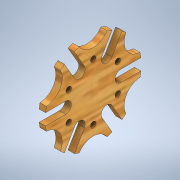
# Autodesk Inventor part: GenevaGear
Saved by Autodesk Inventor 2020.2 (Build 242310000, 310)
## iProperties
Created: 2019-12-15
Part Number: GenevaGear
Material: Plywood, Finish
Document SubType Name: Modeling
Designer: Paul Lefeuvre
Density: 0.552 g/cm^3
Appearance: Plywood - New
Author: Paul Lefeuvre
Autodesk Inventor part; units mm, degrees
ref_plane "YZ Plane" through (0, 0, 0) normal (1, 0, 0) x (0, 1, 0)
ref_plane "XZ Plane" through (0, 0, 0) normal (0, 1, 0) x (-1, 0, 0)
ref_plane "XY Plane" through (0, 0, 0) normal (0, 0, 1) x (1, 0, 0)
sketch "Sketch1" plane through (0, 0, 0) normal (1, 0, 0) x (0, 1, 0)
  circle A0 centre (0, 0) radius 100 construction
  circle A1 centre (0, 0) radius 72.5 construction
  circle A2 centre (0, 0) radius 110 construction
  circle A3 centre (0, 0) radius 67.7492
  line L0 (7.5, -38.8746) -> (7.5, -67.3328) construction
  line L1 (-7.5, -38.8746) -> (-7.5, -67.3328) construction
  arc A4 (7.5, -38.8746) -> (-7.5, -38.8746) centre (0, -38.8746) ccw construction
  line L2 (0, 0) -> (0, -136.3111) construction
  line L3 (8.1, -67.2632) -> (8.1, -38.8746)
  arc A5 (8.1, -38.8746) -> (-8.1, -38.8746) centre (0, -38.8746) ccw
  line L4 (-8.1, -38.8746) -> (-8.1, -67.2632)
  line L5 (62.3017, -26.6168) -> (37.7164, -12.4225)
  arc A6 (37.7164, -12.4225) -> (29.6164, -26.4521) centre (33.6664, -19.4373) ccw
  line L6 (29.6164, -26.4521) -> (54.2017, -40.6464)
  line L7 (54.2017, 40.6464) -> (29.6164, 26.4521)
  arc A7 (29.6164, 26.4521) -> (37.7164, 12.4225) centre (33.6664, 19.4373) ccw
  line L8 (37.7164, 12.4225) -> (62.3017, 26.6168)
  line L9 (-8.1, 67.2632) -> (-8.1, 38.8746)
  arc A8 (-8.1, 38.8746) -> (8.1, 38.8746) centre (0, 38.8746) ccw
  line L10 (8.1, 38.8746) -> (8.1, 67.2632)
  line L11 (-62.3017, 26.6168) -> (-37.7164, 12.4225)
  arc A9 (-37.7164, 12.4225) -> (-29.6164, 26.4521) centre (-33.6664, 19.4373) ccw
  line L12 (-29.6164, 26.4521) -> (-54.2017, 40.6464)
  line L13 (-54.2017, -40.6464) -> (-29.6164, -26.4521)
  arc A10 (-29.6164, -26.4521) -> (-37.7164, -12.4225) centre (-33.6664, -19.4373) ccw
  line L14 (-37.7164, -12.4225) -> (-62.3017, -26.6168)
  line L15 (37.4164, -12.9421) -> (62.0619, -27.1712) construction
  arc A11 (37.4164, -12.9421) -> (29.9164, -25.9325) centre (33.6664, -19.4373) ccw construction
  line L16 (29.9164, -25.9325) -> (54.5619, -40.1616) construction
  circle A12 centre (38.8746, -67.3328) radius 46.3746 construction
  circle A13 centre (38.8746, -67.3328) radius 31.3746 construction
  circle A14 centre (0, 0) radius 31.3746 construction
  arc A15 (49.513, -46.243) -> (15.2911, -66.001) centre (38.8746, -67.3328) ccw
  arc A16 (64.8041, 19.758) -> (64.8041, -19.758) centre (77.7492, 0) ccw
  arc A17 (15.2911, 66.001) -> (49.513, 46.243) centre (38.8746, 67.3328) ccw
  arc A18 (-49.513, 46.243) -> (-15.2911, 66.001) centre (-38.8746, 67.3328) ccw
  arc A19 (-64.8041, -19.758) -> (-64.8041, 19.758) centre (-77.7492, 0) ccw
  arc A20 (-15.2911, -66.001) -> (-49.513, -46.243) centre (-38.8746, -67.3328) ccw
  line L17 (0, 0) -> (144.5472, 0) construction
  circle A21 centre (40, 0) radius 3.9
  circle A22 centre (20, 34.641) radius 3.9
  circle A23 centre (-20, 34.641) radius 3.9
  circle A24 centre (-40, 0) radius 3.9
  circle A25 centre (-20, -34.641) radius 3.9
  circle A26 centre (20, -34.641) radius 3.9
  line L18 (38.8746, -67.3328) -> (33.8746, -58.6725)
  point P0 (-62.3017, 26.6168)
  point P1 (-64.8041, 19.758)
  point P2 (-64.8041, -19.758)
  point P3 (-62.3017, -26.6168)
  point P4 (-49.513, -46.243)
  point P5 (62.3017, -26.6168)
  point P6 (64.8041, -19.758)
  point P7 (64.8041, 19.758)
  point P8 (62.3017, 26.6168)
  point P9 (54.2017, 40.6464)
  point P10 (49.513, 46.243)
  point P11 (15.2911, 66.001)
  point P12 (-15.2911, 66.001)
  point P13 (-49.513, 46.243)
  point P14 (-54.2017, 40.6464)
  dimension "d0" = 200
  dimension "d1" = 145
  dimension "d2" = 220
  dimension "d3" = 7.5
  dimension "d4" = 0.6
  dimension "d7" = 360
  dimension "d11" = 60
  dimension "d13" = 15
  dimension "d18" = 360
  dimension "d22" = 7.8
  dimension "d23" = 40
  dimension "d26" = 360
  dimension "d29" = 10
  constraints: 38 end point, 28 point on circle, 25 centre point, 6 coincident, 4 vertical, 3 tangent, 1 horizontal, 1 parallel, 1 point on line, 113 other
  measures "d0" diameter of A0
  measures "d1" diameter of A1
  measures "d2" diameter of A2
  measures "d3" distance between parallel lines of L0 L2
  measures "d4" distance between parallel lines of L0 L3
  measures "d22" diameter of A21
  measures "d23" distance of A21.centre point (0, 0)
  measures "d29" distance of L18.start L18.end
extrude "Extrusion1" add sketch "Sketch1" along normal blind 9 contours A16 A3 L5 A6 L6 A15 L3 A5 L4 A20 L13 A10 L14 A19 L11 A9 L12 A18 L9 A8 L10 A17 L7 A7 L8
body "Solid1"
